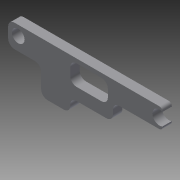
# Autodesk Inventor part: cntrl-space-partA
Saved by Autodesk Inventor 2014 (Build 180170000, 170)
## iProperties
Created: 2014-07-19
Part Number: cntrl-space-partA
Material: Generic
Document SubType Name: Modeling
Designer: james
Density: 1 g/cm^3
Appearance: Default
Author: james
Autodesk Inventor part; units mm, degrees
ref_plane "YZ Plane" through (0, 0, 0) normal (1, 0, 0) x (0, 1, 0)
ref_plane "XZ Plane" through (0, 0, 0) normal (0, 1, 0) x (-1, 0, 0)
ref_plane "XY Plane" through (0, 0, 0) normal (0, 0, 1) x (1, 0, 0)
sketch "Baseline" plane through (0, 0, 0) normal (0, 1, 0) x (-1, 0, 0)
  line L0 (63.1021, -3.4124) -> (14.1385, -3.4124)
  line L1 (14.1385, -3.4124) -> (14.1385, -5.0648)
  line L2 (14.1385, -5.0648) -> (14.1385, -5.0649)
  spline S0 degree 3 poles (14.1385, -5.0649) (14.3614, -4.9411) (14.6142, -4.8646) (14.8873, -4.8646) (15.7454, -4.8646) (16.441, -5.5602) (16.441, -6.4182) (16.441, -7.2763) (15.7454, -7.9719) (14.8873, -7.9719) (14.6143, -7.9719) (14.3615, -7.8953) (14.1385, -7.7716) knots 3 3 3 3 4 4 4 5 5 5 6 6 6 7 7 7 7
  line L3 (14.1385, -5.0649) -> (14.3614, -4.9411) construction
  line L4 (14.3614, -4.9411) -> (14.6142, -4.8646) construction
  line L5 (14.6142, -4.8646) -> (14.8873, -4.8646) construction
  line L6 (14.8873, -4.8646) -> (15.7454, -4.8646) construction
  line L7 (15.7454, -4.8646) -> (16.441, -5.5602) construction
  line L8 (16.441, -5.5602) -> (16.441, -6.4182) construction
  line L9 (16.441, -6.4182) -> (16.441, -7.2763) construction
  line L10 (16.441, -7.2763) -> (15.7454, -7.9719) construction
  line L11 (15.7454, -7.9719) -> (14.8873, -7.9719) construction
  line L12 (14.8873, -7.9719) -> (14.6143, -7.9719) construction
  line L13 (14.6143, -7.9719) -> (14.3615, -7.8953) construction
  line L14 (14.3615, -7.8953) -> (14.1385, -7.7716) construction
  line L15 (14.1385, -7.7716) -> (14.1385, -9.6779)
  line L16 (14.1385, -9.6779) -> (21.9855, -9.6779)
  line L17 (21.9855, -9.6779) -> (29.7235, -9.7124)
  line L18 (29.7235, -9.7124) -> (29.7235, -15.1006)
  line L19 (29.7235, -15.1006) -> (43.3716, -15.1006)
  line L20 (43.3716, -15.1006) -> (43.3716, -19.4875)
  line L21 (43.3716, -19.4875) -> (52.6327, -19.4875)
  line L22 (52.6327, -19.4875) -> (52.6327, -10.7746)
  line L23 (52.6327, -10.7746) -> (63.1149, -10.7746)
  line L24 (63.1149, -10.7746) -> (63.1021, -3.4124)
  spline S1 degree 3 poles (43.4818, -8.1809) (43.4818, -9.7894) (42.1657, -11.1055) (40.5572, -11.1055) knots 0 0 0 0 1 1 1 1
  line L25 (43.4818, -8.1809) -> (43.4818, -9.7894) construction
  line L26 (43.4818, -9.7894) -> (42.1657, -11.1055) construction
  line L27 (42.1657, -11.1055) -> (40.5572, -11.1055) construction
  line L28 (40.5572, -11.1055) -> (34.5316, -11.1055)
  spline S2 degree 3 poles (34.5316, -11.1055) (32.9231, -11.1055) (31.6071, -9.7894) (31.6071, -8.1809) knots 2 2 2 2 3 3 3 3
  line L29 (34.5316, -11.1055) -> (32.9231, -11.1055) construction
  line L30 (32.9231, -11.1055) -> (31.6071, -9.7894) construction
  line L31 (31.6071, -9.7894) -> (31.6071, -8.1809) construction
  line L32 (31.6071, -8.1809) -> (31.6071, -7.7472)
  spline S3 degree 3 poles (31.6071, -7.7472) (31.6071, -6.1387) (32.9231, -4.8227) (34.5316, -4.8227) knots 4 4 4 4 5 5 5 5
  line L33 (31.6071, -7.7472) -> (31.6071, -6.1387) construction
  line L34 (31.6071, -6.1387) -> (32.9231, -4.8227) construction
  line L35 (32.9231, -4.8227) -> (34.5316, -4.8227) construction
  line L36 (34.5316, -4.8227) -> (40.5572, -4.8227)
  spline S4 degree 3 poles (40.5572, -4.8227) (42.1657, -4.8227) (43.4818, -6.1387) (43.4818, -7.7472) knots 6 6 6 6 7 7 7 7
  line L37 (40.5572, -4.8227) -> (42.1657, -4.8227) construction
  line L38 (42.1657, -4.8227) -> (43.4818, -6.1387) construction
  line L39 (43.4818, -6.1387) -> (43.4818, -7.7472) construction
  line L40 (43.4818, -7.7472) -> (43.4818, -8.1809)
  spline S5 degree 3 poles (59.8833, -8.2461) (59.0252, -8.2461) (58.3296, -7.5505) (58.3296, -6.6924) (58.3296, -5.8343) (59.0252, -5.1387) (59.8833, -5.1387) (60.7413, -5.1387) (61.4369, -5.8343) (61.4369, -6.6924) (61.4369, -7.5505) (60.7413, -8.2461) (59.8833, -8.2461) knots 0 0 0 0 1 1 1 2 2 2 3 3 3 4 4 4 4
  line L41 (59.8833, -8.2461) -> (59.0252, -8.2461) construction
  line L42 (59.0252, -8.2461) -> (58.3296, -7.5505) construction
  line L43 (58.3296, -7.5505) -> (58.3296, -6.6924) construction
  line L44 (58.3296, -6.6924) -> (58.3296, -5.8343) construction
  line L45 (58.3296, -5.8343) -> (59.0252, -5.1387) construction
  line L46 (59.0252, -5.1387) -> (59.8833, -5.1387) construction
  line L47 (59.8833, -5.1387) -> (60.7413, -5.1387) construction
  line L48 (60.7413, -5.1387) -> (61.4369, -5.8343) construction
  line L49 (61.4369, -5.8343) -> (61.4369, -6.6924) construction
  line L50 (61.4369, -6.6924) -> (61.4369, -7.5505) construction
  line L51 (61.4369, -7.5505) -> (60.7413, -8.2461) construction
  line L52 (60.7413, -8.2461) -> (59.8833, -8.2461) construction
  line L53 (63.1021, -3.4124) -> (14.1385, -3.4124)
  line L54 (14.1385, -3.4124) -> (14.1385, -5.0648)
  line L55 (14.1385, -5.0648) -> (14.1385, -5.0649)
  spline S6 degree 3 poles (14.1385, -5.0649) (14.3614, -4.9411) (14.6142, -4.8646) (14.8873, -4.8646) (15.7454, -4.8646) (16.441, -5.5602) (16.441, -6.4182) (16.441, -7.2763) (15.7454, -7.9719) (14.8873, -7.9719) (14.6143, -7.9719) (14.3615, -7.8953) (14.1385, -7.7716) knots 3 3 3 3 4 4 4 5 5 5 6 6 6 7 7 7 7
  line L56 (14.1385, -5.0649) -> (14.3614, -4.9411) construction
  line L57 (14.3614, -4.9411) -> (14.6142, -4.8646) construction
  line L58 (14.6142, -4.8646) -> (14.8873, -4.8646) construction
  line L59 (14.8873, -4.8646) -> (15.7454, -4.8646) construction
  line L60 (15.7454, -4.8646) -> (16.441, -5.5602) construction
  line L61 (16.441, -5.5602) -> (16.441, -6.4182) construction
  line L62 (16.441, -6.4182) -> (16.441, -7.2763) construction
  line L63 (16.441, -7.2763) -> (15.7454, -7.9719) construction
  line L64 (15.7454, -7.9719) -> (14.8873, -7.9719) construction
  line L65 (14.8873, -7.9719) -> (14.6143, -7.9719) construction
  line L66 (14.6143, -7.9719) -> (14.3615, -7.8953) construction
  line L67 (14.3615, -7.8953) -> (14.1385, -7.7716) construction
  line L68 (14.1385, -7.7716) -> (14.1385, -9.6779)
  line L69 (14.1385, -9.6779) -> (21.9855, -9.6779)
  line L70 (21.9855, -9.6779) -> (29.7235, -9.7124)
  line L71 (29.7235, -9.7124) -> (29.7235, -15.1006)
  line L72 (29.7235, -15.1006) -> (43.3716, -15.1006)
  line L73 (43.3716, -15.1006) -> (43.3716, -19.4875)
  line L74 (43.3716, -19.4875) -> (52.6327, -19.4875)
  line L75 (52.6327, -19.4875) -> (52.6327, -10.7746)
  line L76 (52.6327, -10.7746) -> (63.1149, -10.7746)
  line L77 (63.1149, -10.7746) -> (63.1021, -3.4124)
  spline S7 degree 3 poles (43.4818, -8.1809) (43.4818, -9.7894) (42.1657, -11.1055) (40.5572, -11.1055) knots 0 0 0 0 1 1 1 1
  line L78 (43.4818, -8.1809) -> (43.4818, -9.7894) construction
  line L79 (43.4818, -9.7894) -> (42.1657, -11.1055) construction
  line L80 (42.1657, -11.1055) -> (40.5572, -11.1055) construction
  line L81 (40.5572, -11.1055) -> (34.5316, -11.1055)
  spline S8 degree 3 poles (34.5316, -11.1055) (32.9231, -11.1055) (31.6071, -9.7894) (31.6071, -8.1809) knots 2 2 2 2 3 3 3 3
  line L82 (34.5316, -11.1055) -> (32.9231, -11.1055) construction
  line L83 (32.9231, -11.1055) -> (31.6071, -9.7894) construction
  line L84 (31.6071, -9.7894) -> (31.6071, -8.1809) construction
  line L85 (31.6071, -8.1809) -> (31.6071, -7.7472)
  spline S9 degree 3 poles (31.6071, -7.7472) (31.6071, -6.1387) (32.9231, -4.8227) (34.5316, -4.8227) knots 4 4 4 4 5 5 5 5
  line L86 (31.6071, -7.7472) -> (31.6071, -6.1387) construction
  line L87 (31.6071, -6.1387) -> (32.9231, -4.8227) construction
  line L88 (32.9231, -4.8227) -> (34.5316, -4.8227) construction
  line L89 (34.5316, -4.8227) -> (40.5572, -4.8227)
  spline S10 degree 3 poles (40.5572, -4.8227) (42.1657, -4.8227) (43.4818, -6.1387) (43.4818, -7.7472) knots 6 6 6 6 7 7 7 7
  line L90 (40.5572, -4.8227) -> (42.1657, -4.8227) construction
  line L91 (42.1657, -4.8227) -> (43.4818, -6.1387) construction
  line L92 (43.4818, -6.1387) -> (43.4818, -7.7472) construction
  line L93 (43.4818, -7.7472) -> (43.4818, -8.1809)
  spline S11 degree 3 poles (59.8833, -8.2461) (59.0252, -8.2461) (58.3296, -7.5505) (58.3296, -6.6924) (58.3296, -5.8343) (59.0252, -5.1387) (59.8833, -5.1387) (60.7413, -5.1387) (61.4369, -5.8343) (61.4369, -6.6924) (61.4369, -7.5505) (60.7413, -8.2461) (59.8833, -8.2461) knots 0 0 0 0 1 1 1 2 2 2 3 3 3 4 4 4 4
  line L94 (59.8833, -8.2461) -> (59.0252, -8.2461) construction
  line L95 (59.0252, -8.2461) -> (58.3296, -7.5505) construction
  line L96 (58.3296, -7.5505) -> (58.3296, -6.6924) construction
  line L97 (58.3296, -6.6924) -> (58.3296, -5.8343) construction
  line L98 (58.3296, -5.8343) -> (59.0252, -5.1387) construction
  line L99 (59.0252, -5.1387) -> (59.8833, -5.1387) construction
  line L100 (59.8833, -5.1387) -> (60.7413, -5.1387) construction
  line L101 (60.7413, -5.1387) -> (61.4369, -5.8343) construction
  line L102 (61.4369, -5.8343) -> (61.4369, -6.6924) construction
  line L103 (61.4369, -6.6924) -> (61.4369, -7.5505) construction
  line L104 (61.4369, -7.5505) -> (60.7413, -8.2461) construction
  line L105 (60.7413, -8.2461) -> (59.8833, -8.2461) construction
  point P0 (0, 0)
  constraints: 68 end point, 34 other
sketch "Sketch2" plane through (0, 0, 0) normal (0, 1, 0) x (-1, 0, 0)
  line L0 (15.1402, -3.4404) -> (61.0861, -3.4404)
  line L1 (63.0861, -5.4404) -> (63.0861, -8.7534)
  line L2 (61.0861, -10.7534) -> (54.6099, -10.7534)
  line L3 (52.6099, -12.7534) -> (52.6099, -17.4949)
  line L4 (50.6099, -19.4949) -> (45.3921, -19.4949)
  line L5 (43.3921, -17.4949) -> (43.3921, -17.1242)
  line L6 (41.3921, -15.1242) -> (31.8442, -15.1242)
  line L7 (29.8442, -13.1242) -> (29.8442, -11.699)
  line L8 (27.8442, -9.699) -> (22.0824, -9.699)
  line L9 (22.0824, -9.699) -> (15.1402, -9.699)
  line L10 (14.1402, -8.699) -> (14.1402, -4.4404)
  circle A0 centre (59.8888, -6.5187) radius 2.0083
  arc A1 (14.1402, -8.527) -> (14.1402, -4.5103) centre (15.0844, -6.5187) ccw
  line L11 (41.3921, -11.2437) -> (33.434, -11.2437)
  line L12 (31.434, -9.2437) -> (31.434, -6.7912)
  line L13 (33.434, -4.7912) -> (41.3921, -4.7912)
  line L14 (43.3921, -6.7912) -> (43.3921, -9.2437)
  arc A2 (33.434, -4.7912) -> (31.434, -6.7912) centre (33.434, -6.7912) ccw
  arc A3 (31.434, -9.2437) -> (33.434, -11.2437) centre (33.434, -9.2437) ccw
  arc A4 (41.3921, -11.2437) -> (43.3921, -9.2437) centre (41.3921, -9.2437) ccw
  arc A5 (43.3921, -6.7912) -> (41.3921, -4.7912) centre (41.3921, -6.7912) ccw
  arc A6 (29.8442, -11.699) -> (27.8442, -9.699) centre (27.8442, -11.699) ccw
  arc A7 (29.8442, -13.1242) -> (31.8442, -15.1242) centre (31.8442, -13.1242) ccw
  arc A8 (43.3921, -17.1242) -> (41.3921, -15.1242) centre (41.3921, -17.1242) ccw
  arc A9 (43.3921, -17.4949) -> (45.3921, -19.4949) centre (45.3921, -17.4949) ccw
  arc A10 (50.6099, -19.4949) -> (52.6099, -17.4949) centre (50.6099, -17.4949) ccw
  arc A11 (54.6099, -10.7534) -> (52.6099, -12.7534) centre (54.6099, -12.7534) ccw
  arc A12 (61.0861, -10.7534) -> (63.0861, -8.7534) centre (61.0861, -8.7534) ccw
  arc A13 (63.0861, -5.4404) -> (61.0861, -3.4404) centre (61.0861, -5.4404) ccw
  arc A14 (15.1402, -3.4404) -> (14.1402, -4.4404) centre (15.1402, -4.4404) ccw
  arc A15 (14.1402, -8.699) -> (15.1402, -9.699) centre (15.1402, -8.699) ccw
  point P0 (0, 0)
  point P1 (14.1402, -3.4404)
  point P2 (63.0861, -3.4404)
  point P3 (63.0861, -10.7534)
  point P4 (52.6099, -10.7534)
  point P5 (52.6099, -19.4949)
  point P6 (43.3921, -19.4949)
  point P7 (43.3921, -15.1242)
  point P8 (29.8442, -15.1242)
  point P9 (29.8442, -9.699)
  point P10 (14.1402, -9.699)
  dimension "d2" = 2
  dimension "d3" = 2
  dimension "d4" = 1
  constraints: 30 end point, 30 point on circle, 28 tangent, 22 point on line, 16 centre point, 11 equal radius, 11 parallel, 2 horizontal, 2 perpendicular, 1 coincident, 1 vertical, 2 other
  measures "d2" radius of A2
  measures "d3" radius of A6
  measures "d4" radius of A14
extrude "Extrusion2" add sketch "Sketch2" along normal blind 3 contours L0 A13 L1 A12 L2 A11 L3 A10 L4 A9 L5 A8 L6 A7 L7 A6 L8 L9 A15 L10 A1 A14
body "Solid2"
